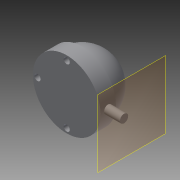
# Autodesk Inventor part: Capteur optoforce
Saved by Autodesk Inventor 2015 (Build 190159000, 159)
## iProperties
Created: 2015-09-16
Part Number: Capteur optoforce
Material: Générique
Document SubType Name: Modeling
Designer: Morgane Dauphin
Density: 1 g/cm^3
Appearance: Par défaut
Author: Morgane Dauphin
Autodesk Inventor part; units mm, degrees
ref_plane "YZ Plane" through (0, 0, 0) normal (1, 0, 0) x (0, 1, 0)
ref_plane "XZ Plane" through (0, 0, 0) normal (0, 1, 0) x (-1, 0, 0)
ref_plane "XY Plane" through (0, 0, 0) normal (0, 0, 1) x (1, 0, 0)
sketch "Esquisse1" plane through (0, 0, 0) normal (0, 1, 0) x (-1, 0, 0)
  circle A0 centre (0, 0) radius 11
  dimension "d1" = 22
  constraints: 1 centre point
  measures "d1" diameter of A0
extrude "Extrusion1" add sketch "Esquisse1" along normal blind 5
sketch "Esquisse2" plane through (0, 5, 0) normal (0, 1, 0) x (1, 0, 0)
  arc A0 (-10, 0) -> (10, 0) centre (0, 0) ccw
  line L0 (-10, 0) -> (10, 0)
  dimension "d4" = 20
  constraints: 2 end point, 2 point on circle, 1 centre point, 1 coincident, 1 horizontal
  measures "d4" diameter of A0
revolve "Révolution1" add sketch "Esquisse2" angle 180 about axis through (-10, 5, 0) along (-1, 0, 0)
ref_plane "Plan de construction1" through (16.1473, 5, 0) normal (1, 0, 0) x (0, 0, -1)
sketch "Esquisse6" plane through (16.1473, 5, 0) normal (1, 0, 0) x (0, 0, -1)
  circle A0 centre (0, -2.5) radius 1.35
  point P0 (0, -5)
  point P1 (0, -1.15)
  dimension "d11" = 2.7
  constraints: 1 vertical alignment, 2 other
extrude "Extrusion4" add sketch "Esquisse6" against normal blind 5.25
sketch "Esquisse7" plane through (0, 0, 0) normal (0, -1, 0) x (1, 0, 0)
  circle A0 centre (0, 9.5) radius 1
  circle A1 centre (0, -9.5) radius 1
  circle A2 centre (-9.5, 0) radius 1
  point P0 (0, 0)
  dimension "d15" = 2
  dimension "d16" = 2
  dimension "d17" = 2
  constraints: 3 centre point
  measures "d15" diameter of A0
  measures "d16" diameter of A2
  measures "d17" diameter of A1
extrude "Extrusion5" cut sketch "Esquisse7" against normal blind 4
